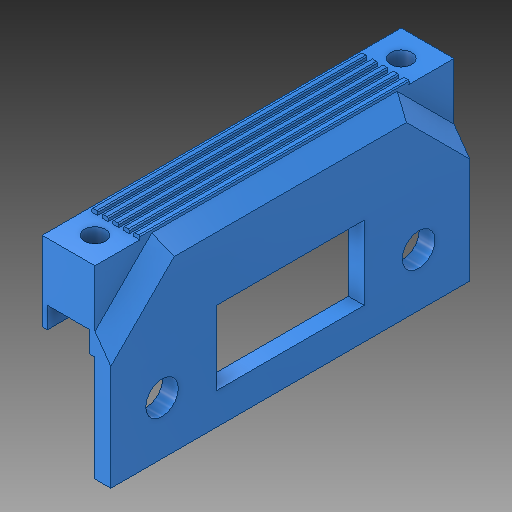
# Autodesk Inventor part: КВ33.044.205 - Держатель ремня
Saved by Autodesk Inventor 2019 (Build 230136000, 136)
## iProperties
Created: 2019-08-18
Part Number: КВ33.044.205 - Держатель ремня
Material: Пластик АБС
Document SubType Name: Modeling
Designer: Петров Иван
Density: 1.06 g/cm^3
Appearance: Голубой
Mass: 12.0412 g
Surface Area: 70.512 cm^2
Volume: 11.3596 cm^3
Author: Петров Иван
Autodesk Inventor part; units mm, degrees
ref_plane "YZ Plane" through (0, 0, 0) normal (1, 0, 0) x (0, 1, 0)
ref_plane "XZ Plane" through (0, 0, 0) normal (0, 1, 0) x (-1, 0, 0)
ref_plane "XY Plane" through (0, 0, 0) normal (0, 0, 1) x (1, 0, 0)
sketch "Эскиз1" plane through (0, 0, 0) normal (1, 0, 0) x (0, 1, 0)
  line L0 (-3, 34) -> (3, 34)
  line L1 (3, 34) -> (3, -34)
  line L2 (3, -34) -> (-3, -34)
  line L3 (-3, -34) -> (-3, 34)
  line L4 (-3, 34) -> (3, -34) construction
  line L5 (3, 34) -> (-3, -34) construction
  line L6 (-3, 34) -> (17, 34)
  line L7 (17, 34) -> (17, 14)
  line L8 (17, 14) -> (-3, 14)
  line L9 (-3, 14) -> (-3, 34)
  line L10 (-3, -34) -> (17, -34)
  line L11 (17, -34) -> (17, -14)
  line L12 (17, -14) -> (-3, -14)
  line L13 (-3, -14) -> (-3, -34)
  point P0 (0, 0)
  dimension "d0" = 6
  dimension "d1" = 68
  dimension "d2" = 20
  dimension "d3" = 20
  dimension "d4" = 20
  dimension "d5" = 20
  constraints: 28 end point, 6 parallel, 3 horizontal, 3 perpendicular, 2 midpoint
  measures "d0" distance of L1.end L2.end
  measures "d1" distance of L0.end L1.end
  measures "d2" distance of L7.end L8.end
  measures "d3" distance of L6.end L7.end
  measures "d4" distance of L12.end L11.end
  measures "d5" distance of L11.end L10.end
extrude "Выдавливание1" add sketch "Эскиз1" along normal blind 3
sketch "Эскиз2" plane through (3, 0, 0) normal (1, 0, 0) x (0, 0, -1)
  line L0 (-14, 17) -> (-34, 17) projected
  line L1 (-34, 17) -> (-24.3, 17)
  line L2 (-24.3, 17) -> (-24.3, 7)
  line L3 (-24.3, 7) -> (-34, 7)
  line L4 (-34, 7) -> (-34, 17)
  line L5 (0, 0) -> (0, 5.665)
  circle A0 centre (-24.3, 7) radius 3.1
  circle A1 centre (24.3, 7) radius 3.1
  dimension "d8" = 9.7
  dimension "d9" = 10
  dimension "d10" = 6.2
  constraints: 10 end point, 2 centre point, 2 parallel, 1 coincident, 1 horizontal, 1 perpendicular, 1 symmetric about line, 1 vertical, 1 other
  measures "d8" distance of L2.end L3.end
  measures "d9" distance of L1.end L2.end
  measures "d10" diameter of A0
extrude "Выдавливание2" cut sketch "Эскиз2" against normal blind 10 contours A0 L3 L2 | L2 L3 A0 | A1
sketch "Эскиз3" plane through (3, 0, 0) normal (1, 0, 0) x (0, 0, -1)
  line L0 (-34, 17) -> (-34, -3) projected
  line L1 (-34, 17) -> (34, 17)
  line L2 (34, 17) -> (34, 32)
  line L3 (34, 32) -> (-34, 32)
  line L4 (-34, 32) -> (-34, 17)
  point P0 (0, 0)
  dimension "d13" = 68
  dimension "d14" = 15
  constraints: 8 end point, 2 parallel, 1 horizontal, 1 perpendicular
  measures "d13" distance of L3.end L2.end
  measures "d14" distance of L1.end L2.end
extrude "Выдавливание3" add sketch "Эскиз3" against normal blind 3
sketch "Эскиз4" plane through (3, 0, 0) normal (1, 0, 0) x (0, 0, -1)
  line L0 (-34, 32) -> (34, 32) projected
  line L1 (-34, 32) -> (-22, 32)
  line L2 (-22, 32) -> (-22, 17)
  line L3 (-22, 17) -> (-34, 17)
  line L4 (-34, 17) -> (-34, 32)
  line L5 (34, 32) -> (22, 32)
  line L6 (22, 32) -> (22, 17)
  line L7 (22, 17) -> (34, 17)
  line L8 (34, 17) -> (34, 32)
  point P0 (0, 0)
  dimension "d17" = 12
  dimension "d18" = 15
  dimension "d19" = 12
  dimension "d20" = 15
  constraints: 16 end point, 4 parallel, 2 horizontal, 2 perpendicular
  measures "d17" distance of L2.end L3.end
  measures "d18" distance of L1.end L2.end
  measures "d19" distance of L7.end L6.end
  measures "d20" distance of L6.end L5.end
extrude "Выдавливание4" cut sketch "Эскиз4" against normal blind 3
chamfer "Фаска1" distance 12 angle 45 2 edges at (1.5, 17, 22) (1.5, 17, -22)
sketch "Эскиз8" plane through (0, 0, 0) normal (-1, 0, 0) x (0, 0, 1)
  line L0 (-22, 32) -> (-22, 29) projected
  line L1 (-22, 32) -> (-3.9189, 32)
  line L2 (-3.9189, 32) -> (-3.9189, 23.986)
  line L3 (-3.9189, 23.986) -> (-22, 23.986)
  line L4 (-22, 23.986) -> (-22, 32)
  line L5 (22, 29) -> (22, 32) projected
  line L6 (22, 29) -> (-4.734, 29)
  line L7 (-4.734, 29) -> (-4.734, 23.986)
  line L8 (-4.734, 23.986) -> (22, 23.986)
  line L9 (22, 23.986) -> (22, 29)
  line L10 (-22, 32) -> (22, 32) projected
  line L11 (-4.734, 23.986) -> (22, 23.986)
  line L12 (22, 23.986) -> (22, 32)
  line L13 (22, 32) -> (-4.734, 32)
  line L14 (-4.734, 32) -> (-4.734, 23.986)
  point P0 (0, 0)
  constraints: 24 end point, 6 parallel, 3 horizontal, 3 perpendicular, 1 point on line
extrude "Выдавливание7" add sketch "Эскиз8" along normal blind 10
sketch "Эскиз9" plane through (0, 0, 0) normal (-1, 0, 0) x (0, 0, 1)
  line L0 (-22, 23.986) -> (-22, 29) projected
  line L1 (-34, -3) -> (-34, 17) projected
  line L2 (-22, 23.986) -> (-34, 23.986)
  line L3 (-34, 23.986) -> (-34, 17.018)
  line L4 (-34, 17.018) -> (-22, 17.018)
  line L5 (-22, 17.018) -> (-22, 23.986)
  line L6 (22, 29) -> (22, 23.986) projected
  line L7 (22, 23.986) -> (34, 23.986)
  line L8 (34, 23.986) -> (34, 17)
  line L9 (34, 17) -> (22, 17)
  line L10 (22, 17) -> (22, 23.986)
  line L11 (22, 32) -> (22, 29) projected
  line L12 (22, 32) -> (34, 32)
  line L13 (34, 32) -> (34, 23.986)
  line L14 (34, 23.986) -> (22, 23.986)
  line L15 (22, 23.986) -> (22, 32)
  line L16 (-22, 29) -> (-22, 32) projected
  line L17 (-22, 32) -> (-34, 32)
  line L18 (-34, 32) -> (-34, 23.986)
  line L19 (-34, 23.986) -> (-22, 23.986)
  line L20 (-22, 23.986) -> (-22, 32)
  point P0 (0, 0)
  dimension "d48" = 6.968
  constraints: 32 end point, 8 parallel, 4 horizontal, 4 perpendicular, 1 point on line
  measures "d48" distance of L3.end L2.end
extrude "Выдавливание8" add sketch "Эскиз9" along normal blind 10
sketch "Эскиз10" plane through (3, 32, 22) normal (0, 1, 0) x (1, 0, 0)
  line L0 (-13, -12) -> (-13, 56) projected
  line L1 (-13, 56) -> (-8, 56)
  line L2 (-8, 56) -> (-8, 51)
  line L3 (-8, 51) -> (-13, 51)
  line L4 (-13, 51) -> (-13, 56)
  circle A0 centre (-8, 51) radius 2
  line L5 (-13, 22) -> (-9.0624, 22)
  circle A1 centre (-8, -7) radius 2
  point P0 (-3, 22)
  dimension "d51" = 5
  dimension "d52" = 5
  dimension "d53" = 4
  constraints: 10 end point, 2 centre point, 2 horizontal, 2 parallel, 1 coincident, 1 midpoint, 1 perpendicular, 1 symmetric about line, 1 other
  measures "d51" distance of L2.end L3.end
  measures "d52" distance of L1.end L2.end
  measures "d53" diameter of A0
extrude "Выдавливание9" cut sketch "Эскиз10" against normal blind 20 contours A0 L2 L3 | L3 L2 A0 | A1
chamfer "Фаска2" distance 3 angle 45 3 edges at (0, 22.9999, 27.9999) (0, 23.009, -27.9909) (3, 32, 0)
sketch "Эскиз11" plane through (0, 32, -34) normal (0, 0, -1) x (-1, 0, 0)
  line L0 (0, -14.982) -> (10, -14.982) projected
  line L1 (5, -14.982) -> (1, -14.982)
  line L2 (1, -14.982) -> (9, -14.982)
  line L3 (9, -14.982) -> (1, -14.982)
  line L4 (1, -14.982) -> (1, -10.982)
  line L5 (1, -10.982) -> (9, -10.982)
  line L6 (9, -10.982) -> (9, -14.982)
  line L7 (9, -14.982) -> (1, -14.982)
  line L8 (1, -14.982) -> (1, -15.7574)
  line L9 (1, -15.7574) -> (9, -15.7574)
  line L10 (9, -15.7574) -> (9, -14.982)
  point P0 (0, -32)
  dimension "d59" = 4
  dimension "d60" = 8
  dimension "d61" = 8
  dimension "d62" = 4
  constraints: 20 end point, 4 parallel, 2 horizontal, 2 perpendicular, 2 point on line, 1 midpoint
  measures "d59" distance of L1.start L1.end
  measures "d60" distance of L1.end L2.end
  measures "d61" distance of L4.end L5.end
  measures "d62" distance of L3.end L4.end
extrude "Выдавливание10" cut sketch "Эскиз11" against normal blind 77.25
sketch "Эскиз15" plane through (-10, 32, -34) normal (0, 1, 0) x (1, 0, 0)
  line L0 (10, -34) -> (10, -8.5)
  line L1 (10, -20) -> (10, -48) projected
  line L2 (10, -8.5) -> (10, -59.5)
  line L3 (10, -59.5) -> (8.86, -59.5)
  line L4 (8.86, -59.5) -> (8.86, -8.5)
  line L5 (8.86, -8.5) -> (10, -8.5)
  line L6 (10, -8.5) -> (10, -59.5)
  line L7 (9.43, -8.5) -> (9.43, -9.1168)
  line L8 (6.86, -8.5) -> (8, -8.5)
  line L9 (8, -8.5) -> (8, -59.5)
  line L10 (8, -59.5) -> (6.86, -59.5)
  line L11 (6.86, -59.5) -> (6.86, -8.5)
  line L12 (7.43, -8.5) -> (7.43, -9.683)
  line L13 (6, -8.5) -> (4.86, -8.5)
  line L14 (4.86, -8.5) -> (4.86, -59.5)
  line L15 (4.86, -59.5) -> (6, -59.5)
  line L16 (6, -59.5) -> (6, -8.5)
  line L17 (5.43, -8.5) -> (5.43, -9.2113)
  line L18 (4, -8.5) -> (2.86, -8.5)
  line L19 (2.86, -8.5) -> (2.86, -59.5)
  line L20 (2.86, -59.5) -> (4, -59.5)
  line L21 (4, -59.5) -> (4, -8.5)
  line L22 (3.43, -8.5) -> (3.43, -9.2465)
  line L23 (2, -8.5) -> (0.86, -8.5)
  line L24 (0.86, -8.5) -> (0.86, -59.5)
  line L25 (0.86, -59.5) -> (2, -59.5)
  line L26 (2, -59.5) -> (2, -8.5)
  line L27 (1.43, -8.5) -> (1.43, -9.3435)
  dimension "d82" = 25.5
  dimension "d83" = 51
  dimension "d84" = 1.14
  dimension "d85" = 51
  dimension "d86" = 1.14
  dimension "d87" = 51
  dimension "d88" = 0
  dimension "d89" = 2
  dimension "d90" = 1.14
  dimension "d91" = 51
  dimension "d92" = 0
  dimension "d93" = 2
  dimension "d94" = 1.14
  dimension "d95" = 51
  dimension "d96" = 0
  dimension "d97" = 2
  dimension "d98" = 1.14
  dimension "d99" = 51
  dimension "d100" = 0
  dimension "d101" = 2
  constraints: 54 end point, 10 parallel, 5 horizontal, 5 midpoint, 5 perpendicular, 5 vertical, 1 collinear, 1 point on line
  measures "d82" distance of L0.start L0.end
  measures "d83" distance of L0.end L2.end
  measures "d84" distance of L4.end L5.end
  measures "d85" distance of L3.end L4.end
  measures "d86" distance of L9.end L10.end
  measures "d87" distance of L8.end L9.end
  measures "d88" distance between parallel lines of L5 L8
  measures "d89" horizontal distance of L7.end L12.end
  measures "d90" distance of L15.end L14.end
  measures "d91" distance of L14.end L13.end
  measures "d92" distance from line of L12.start L13
  measures "d93" horizontal distance of L12.end L17.end
  measures "d94" distance of L20.end L19.end
  measures "d95" distance of L19.end L18.end
  measures "d96" distance between parallel lines of L13 L18
  measures "d97" horizontal distance of L22.end L17.end
  measures "d98" distance of L25.end L24.end
  measures "d99" distance of L24.end L23.end
  measures "d100" distance between parallel lines of L18 L23
  measures "d101" horizontal distance of L22.end L27.end
extrude "Выдавливание12" add sketch "Эскиз15" along normal blind 0.7
chamfer "Фаска3" distance 0.2 angle 45 10 edges at (-1.14, 32.7, 0) (0, 32.7, 0) (-2, 32.7, 0) (-3.14, 32.7, 0) (-5.14, 32.7, 0) (-4, 32.7, 0) (-6, 32.7, 0) (-7.14, 32.7, 0) (-8, 32.7, 0) (-9.14, 32.7, 0)
